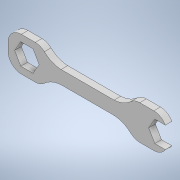
# Autodesk Inventor part: 3_4_inchWrench
Saved by Autodesk Inventor 2020.2 (Build 242310000, 310)
## iProperties
Created: 2019-11-16
Part Number: 3_4_inchWrench
Material: Generic
Document SubType Name: Modeling
Designer: steele
Density: 1 g/cm^3
Appearance: Default
Author: steele
Autodesk Inventor part; units mm, degrees
ref_plane "YZ Plane" through (0, 0, 0) normal (1, 0, 0) x (0, 1, 0)
ref_plane "XZ Plane" through (0, 0, 0) normal (0, 1, 0) x (-1, 0, 0)
ref_plane "XY Plane" through (0, 0, 0) normal (0, 0, 1) x (1, 0, 0)
sketch "Sketch1" plane through (0, 0, 0) normal (0, 0, 1) x (1, 0, 0)
  line L0 (-50.0439, 16.51) -> (-63.5, 16.51)
  line L1 (-76.2, 3.81) -> (-76.2, -3.81)
  line L2 (-76.2, -16.51) -> (76.2, 16.51) construction
  line L3 (76.2, -16.51) -> (-76.2, 16.51) construction
  line L4 (-52.2524, 10.1244) -> (-46.3865, -0.0356)
  line L5 (-46.3865, -0.0356) -> (-52.2524, -10.1956)
  line L6 (-52.2524, -10.1956) -> (-63.9841, -10.1956)
  line L7 (-63.9841, -10.1956) -> (-69.85, -0.0356)
  line L8 (-69.85, -0.0356) -> (-63.9841, 10.1244)
  line L9 (-63.9841, 10.1244) -> (-52.2524, 10.1244)
  line L10 (76.2009, -10.1956) -> (76.2, -10.1972)
  line L11 (74.477, -10.1972) -> (64.4682, -10.1972)
  line L12 (64.4682, -10.1972) -> (58.6024, -0.0372)
  line L13 (58.6024, -0.0372) -> (64.4682, 10.1228)
  line L14 (64.4682, 10.1228) -> (74.5199, 10.1228)
  line L15 (-25.4, -6.35) -> (25.4, -6.35) construction
  line L16 (25.4, -6.35) -> (25.4, 6.35) construction
  line L17 (25.4, 6.35) -> (-25.4, 6.35) construction
  line L18 (-25.4, 6.35) -> (-25.4, -6.35) construction
  line L19 (-25.4, -6.35) -> (25.4, 6.35) construction
  line L20 (25.4, -6.35) -> (-25.4, 6.35) construction
  line L21 (-44.45, 16.51) -> (-44.45, -16.51) construction
  line L22 (44.45, 16.51) -> (44.45, -16.51) construction
  arc A0 (-41.3977, 13.1123) -> (-25.4, 6.35) centre (-24.1053, 31.717) ccw
  arc A1 (-25.4, -6.35) -> (-41.3977, -13.1123) centre (-24.1053, -31.717) ccw
  arc A2 (25.4, 6.35) -> (41.3977, 13.1123) centre (24.1053, 31.717) ccw
  arc A3 (41.3977, -13.1123) -> (25.4, -6.35) centre (24.1053, -31.717) ccw
  line L23 (-25.4, 6.35) -> (25.4, 6.35)
  line L24 (-25.4, -6.35) -> (25.4, -6.35)
  arc A4 (-41.3977, 13.1123) -> (-50.0439, 16.51) centre (-50.0439, 3.81) ccw
  line L25 (-63.5, -16.51) -> (-50.0439, -16.51)
  line L26 (50.0439, -16.51) -> (63.5, -16.51)
  arc A5 (-50.0439, -16.51) -> (-41.3977, -13.1123) centre (-50.0439, -3.81) ccw
  arc A6 (41.3977, -13.1123) -> (50.0439, -16.51) centre (50.0439, -3.81) ccw
  line L27 (50.0439, 16.51) -> (63.5, 16.51)
  arc A7 (50.0439, 16.51) -> (41.3977, 13.1123) centre (50.0439, 3.81) ccw
  arc A8 (41.3977, -13.1123) -> (50.0439, -16.51) centre (50.0439, -3.81) ccw
  arc A9 (-63.5, 16.51) -> (-76.2, 3.81) centre (-63.5, 3.81) ccw
  arc A10 (-76.2, -3.81) -> (-63.5, -16.51) centre (-63.5, -3.81) ccw
  arc A11 (63.5, -16.51) -> (74.477, -10.1972) centre (63.5, -3.81) ccw
  arc A12 (74.5199, 10.1228) -> (63.5, 16.51) centre (63.5, 3.81) ccw
  line L28 (76.2, -10.1972) -> (76.2, -10.1956) construction
  line L29 (76.2, -10.1956) -> (76.2, -10.1972)
  point P0 (0, 0)
  point P1 (-58.1182, -0.0356)
  point P2 (70.3341, -0.0372)
  point P3 (76.2, 6.35)
  point P4 (41.3977, -13.1123)
  point P5 (50.0439, -16.51)
  dimension "totalLength" = 152.4
  dimension "maxWidth" = 33.02
  dimension "boltWidth" = 20.32
  dimension "d3" = 6.35
  dimension "d4" = 20.32
  dimension "handleLength" = 50.8
  dimension "handleWidth" = 12.7
  dimension "endOfHandle" = 44.45
  dimension "d8" = 44.45
  dimension "arcRadius" = 25.4
  dimension "d10" = 25.4
  dimension "d11" = 25.4
  dimension "outerFillet" = 12.7
  dimension "d15" = 12.7
  dimension "d16" = 12.7
  dimension "d17" = 12.7
  constraints: 60 end point, 31 point on circle, 18 tangent, 17 point on line, 13 centre point, 8 equal radius, 7 perpendicular, 6 horizontal, 5 parallel, 4 midpoint, 2 collinear, 1 vertical, 21 other
  measures "totalLength" distance of L2.end L3.end
  measures "maxWidth" distance of L3.end L2.start
  measures "boltWidth" distance between parallel lines of L6 L9
  measures "d3" distance from line of L7.end L1
  measures "d4" distance between parallel lines of L11 L14
  measures "handleLength" distance of L15.start L15.end
  measures "handleWidth" distance of L16.end L15.end
  measures "endOfHandle" distance from line of L22 point (0, 0)
  measures "d8" distance from line of L21 point (0, 0)
  measures "arcRadius" radius of A0
  measures "d10" radius of A1
  measures "d11" radius of A2
  measures "outerFillet" radius of A4
  measures "d15" radius of A5
  measures "d16" radius of A7
  measures "d17" radius of A9
extrude "Extrusion1" add sketch "Sketch1" along normal blind 6.35
equation "\"maxWidth\" = boltWidth + 2 * minWallThickness"
equation "\"boltWidth\" = boltSize + boltGap"
equation "\"d3\" = minWallThickness"
equation "\"d4\" = boltWidth"
equation "\"endOfHandle\" = 0.5 * handleLength + boltSize"
equation "\"d8\" = endOfHandle"
equation "\"d15\" = outerFillet"
equation "\"d16\" = outerFillet"
equation "\"d17\" = outerFillet"
equation "\"d18\" = minWallThickness"
equation "\"minWallThickness\" = 6.35"
equation "\"boltGap\" = 1.27"
equation "\"boltSize\" = 19.05"
body "Solid1"
